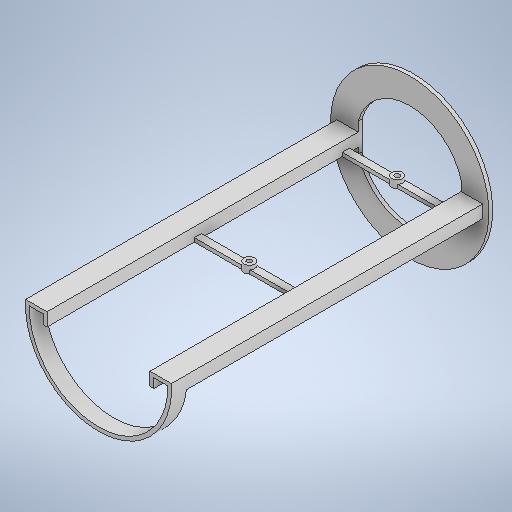
# Autodesk Inventor part: Revised Mount
Saved by Autodesk Inventor 2025 (Build 290162010, 162A)
## iProperties
Created: 2024-06-12
Part Number: Revised Mount
Material: Generic
Document SubType Name: Modeling
Designer: vncnt
Density: 1 g/cm^3
Appearance: Default
Author: vncnt
Autodesk Inventor part; units mm, degrees
ref_plane "YZ Plane" through (0, 0, 0) normal (1, 0, 0) x (0, 1, 0)
ref_plane "XZ Plane" through (0, 0, 0) normal (0, 1, 0) x (-1, 0, 0)
ref_plane "XY Plane" through (0, 0, 0) normal (0, 0, 1) x (1, 0, 0)
sketch "Sketch1" plane through (0, 0, 0) normal (0, 0, 1) x (1, 0, 0)
  circle A0 centre (0, 0) radius 38.75
  dimension "d0" = 77.5
  constraints: 1 centre point, 1 coincident
  measures "d0" diameter of A0
extrude "Extrusion1" add sketch "Sketch1" along normal blind 165.1
sketch "Sketch2" plane through (0, 0, 165.1) normal (0, 0, 1) x (1, 0, 0)
  line L0 (-27.305, -2.5) -> (27.305, -2.5)
  line L1 (27.305, -2.5) -> (27.305, 2.5)
  line L2 (27.305, 2.5) -> (-27.305, 2.5)
  line L3 (-27.305, 2.5) -> (-27.305, -2.5)
  line L4 (-27.305, -2.5) -> (27.305, 2.5) construction
  line L5 (27.305, -2.5) -> (-27.305, 2.5) construction
  line L6 (0, 2.5) -> (41.5863, 2.5)
  line L7 (41.5863, 2.5) -> (41.5863, 42.5)
  line L8 (41.5863, 42.5) -> (0, 42.5)
  line L9 (0, 42.5) -> (0, 2.5)
  line L10 (0, 42.5) -> (-50, 42.5)
  line L11 (-50, 42.5) -> (-50, 2.5)
  line L12 (-50, 2.5) -> (0, 2.5)
  line L13 (0, 2.5) -> (0, 42.5)
  point P0 (0, 0)
  point P1 (-27.305, 2.5)
  dimension "d3" = 54.61
  dimension "d4" = 5
  constraints: 28 end point, 6 parallel, 3 midpoint, 3 perpendicular, 2 horizontal, 1 point on line
  measures "d3" distance of L2.end L1.end
  measures "d4" distance of L2.end L0.start
extrude "Extrusion2" cut sketch "Sketch2" against normal through all
sketch "Sketch3" plane through (0, 0, 0) normal (0, 0, -1) x (-1, 0, 0)
  circle A0 centre (0, 0) radius 42
  constraints: 1 centre point, 1 coincident
extrude "Extrusion3" add sketch "Sketch3" along normal blind 2
sketch "Sketch4" plane through (-27.305, -2.5, 165.1) normal (0, 1, 0) x (1, 0, 0)
  line L0 (0, 165.1) -> (54.61, 165.1) projected
  line L1 (0, 0) -> (0, 165.1) projected
  point P0 (27.305, 165.1)
  point P1 (27.305, 158.496)
  dimension "d9" = 6.604
  dimension "d10" = 27.305
  measures "d9" distance from line of L0 point (27.305, 158.496)
  measures "d10" distance from line of L1 point (27.305, 158.496)
hole "Hole1" at (0, -2.5, 6.604) direction (0, -1, 0) diameter 2.6416 depth 10.979 thread size "6-32 UNC" class "2B" standard "ANSI Unified Screw Threads"
sketch "Sketch5" plane through (-27.305, -2.5, 165.1) normal (0, 1, 0) x (1, 0, 0)
  line L0 (0, 165.1) -> (54.61, 165.1) projected
  line L1 (0, 0) -> (0, 165.1) projected
  point P0 (27.305, 165.1)
  point P1 (27.305, 80.01)
  dimension "d18" = 85.09
  dimension "d26" = 27.305
  measures "d18" distance from line of L0 point (27.305, 80.01)
  measures "d26" distance from line of L1 point (27.305, 80.01)
hole "Hole2" at (0, -2.5, 85.09) direction (0, -1, 0) diameter 2.6416 depth 10.979 thread size "6-32 UNC" class "2B" standard "ANSI Unified Screw Threads"
shell "Shell1" thickness 2 removed faces 1 at (1.4054, -14.5066, 165.1)
sketch "Sketch6" plane through (27.305, 2.5, 165.1) normal (0, 1, 0) x (1, 0, 0)
  circle A0 centre (-27.305, 158.496) radius 1.3208 projected
  circle A1 centre (-27.305, 80.01) radius 1.3208 projected
  line L0 (0, 79.02) -> (0, 81)
  line L1 (-54.61, 81) -> (-54.61, 79.02)
  line L2 (0, 160.401) -> (0, 156.591)
  line L3 (-54.61, 156.591) -> (-54.61, 160.401)
  line L4 (-54.61, 160.401) -> (0, 156.591) construction
  line L5 (0, 160.401) -> (-54.61, 156.591) construction
  line L6 (0, 78.105) -> (0, 81.915)
  line L7 (-54.61, 81.915) -> (-54.61, 78.105)
  line L8 (-54.61, 78.105) -> (0, 81.915) construction
  line L9 (0, 78.105) -> (-54.61, 81.915) construction
  line L10 (-54.61, 165.1) -> (0, 165.1)
  line L11 (0, 165.1) -> (0, 0)
  line L12 (0, 0) -> (-54.61, 0)
  line L13 (-54.61, 0) -> (-54.61, 165.1)
  arc A2 (-25.1118, 160.401) -> (-29.4982, 160.401) centre (-27.305, 158.496) ccw
  arc A3 (-29.4982, 156.591) -> (-25.1118, 156.591) centre (-27.305, 158.496) ccw
  line L14 (-54.61, 160.401) -> (-29.4982, 160.401)
  line L15 (-25.1118, 160.401) -> (0, 160.401)
  line L16 (0, 156.591) -> (-25.1118, 156.591)
  line L17 (-29.4982, 156.591) -> (-54.61, 156.591)
  line L18 (0, 81.915) -> (-25.1118, 81.915)
  line L19 (-29.4982, 81.915) -> (-54.61, 81.915)
  line L20 (-54.61, 78.105) -> (-29.4982, 78.105)
  line L21 (-25.1118, 78.105) -> (0, 78.105)
  arc A4 (-25.1118, 81.915) -> (-29.4982, 81.915) centre (-27.305, 80.01) ccw
  arc A5 (-29.4982, 78.105) -> (-25.1118, 78.105) centre (-27.305, 80.01) ccw
  point P0 (-27.305, 165.1)
  constraints: 44 end point, 13 parallel, 8 point on circle, 5 horizontal, 5 perpendicular, 4 centre point, 4 midpoint, 2 coincident, 1 point on line
extrude "Extrusion4" cut sketch "Sketch6" against normal blind 12.5 contours L11 L12 L13 L20 A5 L21 | L18 A4 L19 L13 L17 A3 L16 L11 | L15 A2 L14 L13 L10 L11
sketch "Sketch7" plane through (0, 0, 0) normal (1, 0, 0) x (0, 1, 0)
  line L0 (-4.5, 165.1) -> (-4.5, 0) projected
  line L1 (-4.5, 0) -> (-49, 0)
  line L2 (0.5, 0) -> (-4.5, 0) projected
  line L3 (-4.5, 0) -> (-55.1519, 0)
  line L4 (-55.1519, 0) -> (-55.1519, 156.9376)
  line L5 (-55.1519, 156.9376) -> (-4.5, 156.9376)
  line L6 (-4.5, 156.9376) -> (-4.5, 0)
  line L7 (-4.5, 0) -> (-56.1519, 0)
  line L8 (-56.1519, 0) -> (-56.1519, 0)
  line L9 (-56.1519, 0) -> (-4.5, 0)
  line L10 (-4.5, 0) -> (-4.5, 0)
  point P0 (0, 0)
  point P1 (-4.5, 156.9376)
  point P2 (-55.1519, 1)
  point P3 (-4.5, 0)
  constraints: 18 end point, 4 equal length, 3 horizontal, 2 perpendicular, 1 point on line
extrude "Extrusion5" cut sketch "Sketch7" along normal through all both and the other way through all
sketch "Sketch9" plane through (0, 0, 0) normal (0, 0, 1) x (1, 0, 0)
  line L0 (-27.305, -4.5) -> (-27.305, 2.5) projected
  line L1 (-27.305, -1) -> (-27.305, 7.524)
  line L2 (-27.305, -4.5) -> (-27.305, -7.524)
  line L3 (27.305, 2.5) -> (27.305, -4.5) projected
  line L4 (27.305, -1) -> (27.305, 7.524)
  line L5 (27.305, 7.524) -> (27.305, -7.524)
  arc A0 (-27.305, -7.524) -> (27.305, -7.524) centre (0, 0) ccw
  arc A1 (27.305, 7.524) -> (-27.305, 7.524) centre (0, 0) ccw
  point P0 (-27.305, 2.5)
  constraints: 8 end point, 4 point on circle, 3 vertical, 2 centre point, 2 midpoint, 1 coincident
extrude "Extrusion7" cut sketch "Sketch9" against normal blind 2.5
sketch "Sketch14" plane through (2.1932, -2.5, 86.995) normal (0, 1, 0) x (1, 0, 0)
  circle A0 centre (-2.1932, 80.391) radius 1.3208 projected
  circle A1 centre (-2.1932, 80.391) radius 1.3208
  circle A2 centre (-2.1932, 80.391) radius 2.905
  circle A3 centre (-2.1932, 1.905) radius 1.3208 projected
  circle A4 centre (-2.1932, 1.905) radius 1.3208
  circle A5 centre (-2.1932, 1.905) radius 2.905
  point P0 (-2.1932, 86.995)
  constraints: 4 centre point, 4 coincident
extrude "Extrusion10" add sketch "Sketch14" along normal blind 2
body "Solid1"
